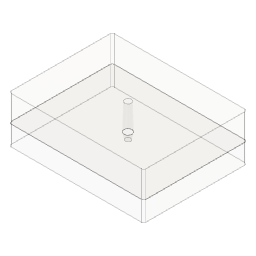
koma (Autodesk Fusion 360 archive; units mm, degrees)
design "MoldSample"
Autodesk Fusion 360 part; units mm, degrees
sketch "スケッチ7" plane through (0, 0, 0) normal (0, 0, 1) x (1, 0, 0)
  line L0 (-40, -25) -> (40, -25)
  line L1 (40, -25) -> (40, 25)
  line L2 (40, 25) -> (-40, 25)
  line L3 (-40, 25) -> (-40, -25)
  line L4 (-40, -25) -> (40, 25) construction
  line L5 (40, -25) -> (-40, 25) construction
  line L6 (-40, 0) -> (40, 0) construction
  line L7 (0, -25) -> (0, 25) construction
  circle A0 centre (-35, 20) radius 2.75
  circle A1 centre (35, 20) radius 2.75
  circle A2 centre (-35, -20) radius 2.75
  circle A3 centre (35, -20) radius 2.75
  line L8 (-29, -23) -> (29, -23)
  line L9 (30, -22) -> (30, 22)
  line L10 (29, 23) -> (-29, 23)
  line L11 (-30, 22) -> (-30, -22)
  line L12 (-30, -23) -> (30, 23) construction
  line L13 (30, -23) -> (-30, 23) construction
  arc A4 (-29, 23) -> (-30, 22) centre (-29, 22) ccw
  arc A5 (30, 22) -> (29, 23) centre (29, 22) ccw
  arc A6 (29, -23) -> (30, -22) centre (29, -22) ccw
  arc A7 (-30, -22) -> (-29, -23) centre (-29, -22) ccw
  circle A8 centre (0, 0) radius 1.5
  arc A9 (-6, 23) -> (6, 23) centre (0, 23) ccw
  arc A10 (-30, -8) -> (-30, 8) centre (-30, 0) ccw
  arc A11 (6, -23) -> (-6, -23) centre (0, -23) ccw
  arc A12 (30, 8) -> (30, -8) centre (30, 0) ccw
  dimension "d41" = 50
  dimension "d42" = 80
  dimension "d43" = 5.5
  dimension "d44" = 5
  dimension "d45" = 5
  dimension "d186" = 46
  dimension "d187" = 10
  dimension "d188" = 1
  dimension "d197" = 3
  dimension "d229" = 8
  dimension "d230" = 6
  constraint horizontal L0
  constraint perpendicular L0 L1
  constraint parallel L0 L2
  constraint parallel L1 L3
  constraint coincident L4 A8.centre
  constraint coincident L5 A8.centre
  constraint coincident A8.centre origin
  constraint midpoint L3 L6.start
  constraint midpoint L1 L6.end
  constraint midpoint L0 L7.start
  constraint midpoint L2 L7.end
  constraint symmetric L7 A0 A1
  constraint symmetric L6 A0 A2
  constraint symmetric L6 A1 A3
  constraint horizontal L8
  constraint perpendicular L8 L9
  constraint parallel L8 L10
  constraint parallel L9 L11
  constraint coincident L12 A8.centre
  constraint coincident L13 A8.centre
  constraint coincident L13.end L11
  constraint coincident L13.end L10
  constraint tangent L11 A4
  constraint tangent L10 A4
  constraint coincident L12.end L10
  constraint coincident L12.end L9
  constraint tangent L10 A5
  constraint tangent L9 A5
  constraint equal A4 A5
  constraint coincident L13.start L9
  constraint coincident L13.start L8
  constraint tangent L9 A6
  constraint tangent L8 A6
  constraint equal A4 A6
  constraint coincident L12.start L8
  constraint coincident L12.start L11
  constraint tangent L8 A7
  constraint tangent L11 A7
  constraint equal A4 A7
  constraint coincident L10 A9.start
  constraint midpoint L10 A9.centre
  constraint coincident L11 A10.start
  constraint midpoint L11 A10.centre
  constraint symmetric L6 A9.start A11.end
  constraint symmetric L6 A9.end A11.start
  constraint symmetric L6 A9 A11
  constraint symmetric L7 A10.start A12.end
  constraint symmetric L7 A10.end A12.start
  constraint symmetric L7 A10 A12
  measures "d41" distance of L0 L2
  measures "d42" distance of L1 L3
  measures "d43" diameter of A0
  measures "d44" distance of L2 A0.centre
  measures "d45" distance of L3 A0.centre
  measures "d186" distance of L8 L10
  measures "d187" distance of L3 L11
  measures "d188" radius of A4
  measures "d197" diameter of A8
  measures "d229" radius of A10
  measures "d230" radius of A9
sketch "Runner" plane through (0, 0, 0) normal (0, 0, 1) x (1, 0, 0)
  line L0 (-14.6, 1.8) -> (-14.6, -1.8)
  arc A0 (-23, -0.6) -> (-21.8, -1.8) centre (-21.8, -0.6) ccw
  line L1 (-17, 1.8) -> (17, 1.8) construction
  line L2 (-14.6, 1.8) -> (-15.4, 3.5)
  line L3 (-17, -3.5) -> (-17, 3.5)
  line L4 (17, 1.8) -> (-17, -1.8) construction
  line L5 (0, 1.8) -> (0, -1.8) construction
  line L6 (-17, 3.5) -> (-15.4, 3.5)
  line L7 (-17, -1.8) -> (-17, 1.8)
  line L8 (-25, -3.5) -> (-9, -3.5) construction
  line L9 (-25.0006, 3.5) -> (-8.9994, 3.5) construction
  arc A1 (21.8, -1.8) -> (23, -0.6) centre (21.8, -0.6) ccw
  line L10 (-17, 1.8) -> (17, -1.8) construction
  line L11 (21.8, -1.8) -> (17, -1.8)
  line L12 (17, 1.8) -> (17, -1.8)
  line L13 (-17, 0) -> (17.3464, 0)
  line L14 (17, 0) -> (23, 0)
  line L15 (-17, 0) -> (-23, 0)
  line L16 (-14.6, -1.8) -> (-15.4, -3.5)
  line L17 (23, 0) -> (23, -0.6)
  line L18 (-17, -3.5) -> (-15.4, -3.5)
  line L19 (-15.4, -3.5) -> (-15.4, 3.5)
  line L20 (17, -1.8) -> (-17, -1.8)
  line L21 (-17, -1.8) -> (-17, 0)
  line L22 (-21.8, -1.8) -> (-17, -1.8)
  line L23 (-23, 0) -> (-23, -0.6)
  circle A2 centre (0, 0) radius 1.8
  circle A3 centre (0, 0) radius 1.5
  dimension "d202" = 1.6
  dimension "d204" = 0.8
  dimension "d210" = 6
  dimension "d211" = 1.2
  dimension "d212" = 3.5
  dimension "d213" = 3.5
  dimension "d214" = 3
  dimension "d215" = 3.6
  dimension "d216" = 17
  constraint horizontal L13
  constraint horizontal L1
  constraint perpendicular L1 L12
  constraint parallel L1 L20
  constraint parallel L7 L12
  constraint coincident A2.centre L10
  constraint coincident A2.centre L4
  constraint midpoint L13.start L7
  constraint vertical L3
  constraint collinear L3 L7
  constraint midpoint L13.start L3
  constraint midpoint L3.end L9
  constraint coincident L2.end L9
  constraint perpendicular L9 L19
  constraint coincident L16.end L8
  constraint coincident L0.end L20
  constraint coincident L16.end L19
  constraint symmetric L0.end L0.start L13
  constraint symmetric L16.end L2.end L13
  constraint horizontal L15
  constraint vertical L23
  constraint horizontal L22
  constraint vertical L21
  constraint collinear L20 L22
  constraint tangent A0 L23
  constraint tangent A0 L22
  constraint midpoint L5.start L1
  constraint midpoint L5.end L20
  constraint symmetric L14.start L13.start L5
  constraint symmetric L15.end L14.end L5
  constraint symmetric L10.end L4.end L5
  constraint symmetric A1.end A0.start L5
  constraint symmetric A1.start A0.end L5
  constraint symmetric A0 L5 A1
  constraint coincident A2.centre A3.centre
  constraint tangent L20 A2
  measures "d202" distance of L3 L19
  measures "d204" distance of L0.end L19
  measures "d210" distance of L3 L23
  measures "d211" radius of A0
  measures "d212" distance of L8 L13
  measures "d213" distance of L9 L13
  measures "d214" diameter of A3
  measures "d215" diameter of A2
  measures "d216" distance of L3 A2.centre
sketch "スケッチ1" plane through (0, 0, 0) normal (0, 0, 1) x (1, 0, 0)
  line L0 (8.5, -3) -> (25.5, -3)
  line L1 (26, -3.5) -> (26, -20.5)
  line L2 (25.5, -21) -> (8.5, -21)
  line L3 (8, -20.5) -> (8, -3.5)
  line L4 (17, -3) -> (17, -21) construction
  line L5 (8, -12) -> (26, -12) construction
  arc A0 (8.5, -3) -> (8, -3.5) centre (8.5, -3.5) ccw
  arc A1 (26, -3.5) -> (25.5, -3) centre (25.5, -3.5) ccw
  arc A2 (25.5, -21) -> (26, -20.5) centre (25.5, -20.5) ccw
  arc A3 (8, -20.5) -> (8.5, -21) centre (8.5, -20.5) ccw
  line L6 (9.7, -4.2) -> (24.3, -4.2)
  line L7 (9.2, -19.3) -> (9.2, -4.7)
  line L8 (24.3, -19.8) -> (9.7, -19.8)
  line L9 (24.8, -4.7) -> (24.8, -19.3)
  arc A4 (9.7, -4.2) -> (9.2, -4.7) centre (9.7, -4.7) ccw
  arc A5 (9.2, -19.3) -> (9.7, -19.8) centre (9.7, -19.3) ccw
  arc A6 (24.3, -19.8) -> (24.8, -19.3) centre (24.3, -19.3) ccw
  arc A7 (24.8, -4.7) -> (24.3, -4.2) centre (24.3, -4.7) ccw
  circle A8 centre (17, -12.03) radius 2.7
  line L10 (14.3525, -11.5) -> (19.6475, -11.5) construction
  line L11 (14.3525, -12.5) -> (19.6475, -12.5) construction
  line L12 (16.5, -9.3767) -> (16.5, -14.6833) construction
  line L13 (17.5, -9.3767) -> (17.5, -14.6833) construction
  line L14 (16.5, -11.5) -> (14.5202, -11.5)
  line L15 (14.5202, -12.5) -> (14.5202, -11.5)
  line L16 (14.5202, -12.5) -> (16.5, -12.5)
  line L17 (15.0202, -11.5) -> (15.0202, -12.5)
  line L18 (16.5, -12.5) -> (16.5, -14.4798)
  line L19 (17.5, -14.4798) -> (17.5, -12.5)
  line L20 (16.5, -13.9798) -> (17.5, -13.9798)
  line L21 (17.5, -14.4798) -> (16.5, -14.4798)
  line L22 (17.5, -12.5) -> (19.4798, -12.5)
  line L23 (19.4798, -11.5) -> (17.5, -11.5)
  line L24 (18.9798, -12.5) -> (18.9798, -11.5)
  line L25 (19.4798, -11.5) -> (19.4798, -12.5)
  line L26 (17.5, -11.5) -> (17.5, -9.5202)
  line L27 (16.5, -9.5202) -> (16.5, -11.5)
  line L28 (17.5, -10.0202) -> (16.5, -10.0202)
  line L29 (16.5, -9.5202) -> (17.5, -9.5202)
  circle A9 centre (13.2, -15.7) radius 1.25
  circle A10 centre (20.8, -15.7) radius 1.25
  point P0 (8, -3)
  point P1 (8, -21)
  point P2 (14.3002, -12)
  point P3 (17, -12)
  dimension "d326" = 18
  dimension "d327" = 18
  dimension "d328" = 8
  dimension "d329" = 3
  dimension "d330" = 0.5
  dimension "d332" = 0.5
  dimension "d333" = 0.03
  dimension "d334" = 5.4
  dimension "d335" = 1.2
  dimension "d336" = 1.2
  dimension "d337" = 1
  dimension "d338" = 1
  dimension "d339" = 0.22
  dimension "d341" = 0.5
  dimension "d343" = 360
  dimension "d366" = 2.5
  dimension "d367" = 12.7
  dimension "d368" = 5.2
  constraint horizontal L0
  constraint vertical L1
  constraint horizontal L2
  constraint vertical L3
  constraint coincident L3 L5.start
  constraint coincident L0 L4.start
  constraint coincident P0 L3
  constraint coincident P0 L0
  constraint tangent L3 A0
  constraint tangent L0 A0
  constraint coincident L1 L5.end
  constraint tangent L0 A1
  constraint tangent L1 A1
  constraint equal A0 A1
  constraint coincident L2 L4.end
  constraint tangent L1 A2
  constraint tangent L2 A2
  constraint equal A0 A2
  constraint coincident P1 L2
  constraint coincident P1 L3
  constraint tangent L2 A3
  constraint tangent L3 A3
  constraint equal A0 A3
  constraint parallel L0 L6
  constraint parallel L3 L7
  constraint parallel L2 L8
  constraint parallel L1 L9
  constraint tangent L6 A4
  constraint tangent L7 A4
  constraint tangent L7 A5
  constraint tangent L8 A5
  constraint equal A4 A5
  constraint tangent L8 A6
  constraint tangent L9 A6
  constraint equal A4 A6
  constraint tangent L9 A7
  constraint tangent L6 A7
  constraint equal A4 A7
  constraint coincident L4 A8.centre
  constraint vertical L4
  constraint horizontal L5
  constraint midpoint L4 L5
  constraint symmetric L5 L6 L8
  constraint symmetric L4 L7 L9
  constraint coincident A8 L10.start
  constraint coincident A8 L10.end
  constraint perpendicular L4 L10
  constraint symmetric L5 L10.start L11.start
  constraint symmetric L5 L10.end L11.end
  constraint coincident A8 L12.start
  constraint coincident A8 L12.end
  constraint vertical L12
  constraint symmetric L4 L12.start L13.start
  constraint symmetric L4 L12.end L13.end
  constraint coincident L10 L14.start
  constraint coincident L12 L14.start
  constraint coincident L10 L14.end
  constraint perpendicular L12 L14
  constraint coincident L11 L15.start
  constraint coincident L12 L16.end
  constraint coincident L11 L16.end
  constraint coincident L5 P2
  constraint coincident A8 P2
  constraint perpendicular L5 L15
  constraint coincident L14 L17.start
  constraint coincident L11 L17.end
  constraint perpendicular L11 L17
  constraint midpoint L4 P3
  constraint symmetric L4 A9 A10
  measures "d326" distance of P0 P1
  measures "d327" distance of L1 L3
  measures "d328" horizontal distance of P0 origin
  measures "d329" vertical distance of P0 origin
  measures "d330" radius of A0
  measures "d332" radius of A4
  measures "d333" distance of L5 A8.centre
  measures "d334" diameter of A8
  measures "d335" distance of L2 L8
  measures "d336" distance of L1 L9
  measures "d337" distance of L10 L11
  measures "d338" distance of L12 L13
  measures "d339" distance of L15 P2
  measures "d341" distance of L15 L17
  measures "d366" diameter of A9
  measures "d367" distance of L0 A9.centre
  measures "d368" distance of L3 A9.centre
ref_plane "作業平面1" through (0, 0, 7.5) normal (0, 0, 1) x (1, 0, 0)
sketch "スケッチ2" plane through (0, 0, 7.5) normal (0, 0, 1) x (1, 0, 0)
  line L0 (8.5, -3) -> (25.5, -3) construction
  line L1 (8, -20.5) -> (8, -3.5) construction
  line L2 (25.5, -21) -> (8.5, -21) construction
  line L3 (26, -3.5) -> (26, -20.5) construction
  arc A0 (26, -3.5) -> (25.5, -3) centre (25.5, -3.5) ccw construction
  arc A1 (8.5, -3) -> (8, -3.5) centre (8.5, -3.5) ccw construction
  arc A2 (8, -20.5) -> (8.5, -21) centre (8.5, -20.5) ccw construction
  arc A3 (25.5, -21) -> (26, -20.5) centre (25.5, -20.5) ccw construction
  line L4 (17, -3) -> (17, -21) construction
  line L5 (8, -12) -> (26, -12) construction
  line L6 (12, -18) -> (22, -18)
  line L7 (23, -17) -> (23, -7)
  line L8 (22, -6) -> (12, -6)
  line L9 (11, -7) -> (11, -17)
  line L10 (11, -18) -> (23, -6) construction
  line L11 (23, -18) -> (11, -6) construction
  arc A4 (12, -6) -> (11, -7) centre (12, -7) ccw
  arc A5 (23, -7) -> (22, -6) centre (22, -7) ccw
  arc A6 (22, -18) -> (23, -17) centre (22, -17) ccw
  arc A7 (11, -17) -> (12, -18) centre (12, -17) ccw
  point P0 (17, -12)
  dimension "d396" = 12
  dimension "d397" = 12
  dimension "d398" = 1
  constraint midpoint L0 L4.start
  constraint midpoint L2 L4.end
  constraint midpoint L1 L5.start
  constraint midpoint L3 L5.end
  constraint horizontal L6
  constraint perpendicular L6 L7
  constraint parallel L6 L8
  constraint parallel L7 L9
  constraint coincident L10 P0
  constraint coincident L11 P0
  constraint midpoint L4 P0
  constraint coincident L11.end L9
  constraint coincident L11.end L8
  constraint tangent L9 A4
  constraint tangent L8 A4
  constraint coincident L10.end L8
  constraint coincident L10.end L7
  constraint tangent L8 A5
  constraint tangent L7 A5
  constraint equal A4 A5
  constraint coincident L11.start L7
  constraint coincident L11.start L6
  constraint tangent L7 A6
  constraint tangent L6 A6
  constraint equal A4 A6
  constraint coincident L10.start L6
  constraint coincident L10.start L9
  constraint tangent L6 A7
  constraint tangent L9 A7
  constraint equal A4 A7
  measures "d396" distance of L7 L9
  measures "d397" distance of L6 L8
  measures "d398" radius of A4
ref_plane "作業平面4" through (0, 0, 6.3) normal (0, 0, 1) x (1, 0, 0)
sketch "スケッチ8" plane through (0, 0, 6.3) normal (0, 0, 1) x (1, 0, 0)
  line L0 (11, -7) -> (11, -17) construction
  line L1 (22, -6) -> (12, -6) construction
  arc A0 (12, -6) -> (11, -7) centre (12, -7) ccw construction
  arc A1 (11, -17) -> (12, -18) centre (12, -17) ccw construction
  line L2 (12, -18) -> (22, -18) construction
  line L3 (23, -17) -> (23, -7) construction
  arc A2 (23, -7) -> (22, -6) centre (22, -7) ccw construction
  arc A3 (22, -18) -> (23, -17) centre (22, -17) ccw construction
  line L4 (21.5, -7) -> (12.5, -7)
  line L5 (12, -7.5) -> (12, -16.5)
  line L6 (12.5, -17) -> (21.5, -17)
  line L7 (22, -16.5) -> (22, -7.5)
  arc A4 (12.5, -7) -> (12, -7.5) centre (12.5, -7.5) ccw
  arc A5 (22, -7.5) -> (21.5, -7) centre (21.5, -7.5) ccw
  arc A6 (21.5, -17) -> (22, -16.5) centre (21.5, -16.5) ccw
  arc A7 (12, -16.5) -> (12.5, -17) centre (12.5, -16.5) ccw
  line L8 (17, -6) -> (17, -18) construction
  line L9 (11, -12) -> (23, -12) construction
  dimension "d400" = 0.5
  dimension "d401" = 1
  dimension "d402" = 1
  constraint parallel L1 L4
  constraint parallel L0 L5
  constraint parallel L2 L6
  constraint parallel L3 L7
  constraint tangent L5 A4
  constraint tangent L4 A4
  constraint tangent L4 A5
  constraint tangent L7 A5
  constraint equal A4 A5
  constraint tangent L7 A6
  constraint tangent L6 A6
  constraint equal A4 A6
  constraint tangent L6 A7
  constraint tangent L5 A7
  constraint equal A4 A7
  constraint midpoint L1 L8.start
  constraint midpoint L2 L8.end
  constraint midpoint L0 L9.start
  constraint midpoint L3 L9.end
  constraint symmetric L5 L7 L8
  constraint symmetric L4 L6 L9
  measures "d400" radius of A4
  measures "d401" distance of L3 L7
  measures "d402" distance of L1 L4
ref_plane "作業平面10" through (0, -12, 0) normal (0, 1, 0) x (0, 0, 1)
sketch "スケッチ28" plane through (0, -12, 0) normal (0, 1, 0) x (1, 0, 0)
  line L0 (17, -7.5) -> (17, 0) construction
  arc A0 (22, -6.3) -> (24.8, 0) centre (7.2558, 4.0252) ccw
  arc A1 (9.2, 0) -> (12, -6.3) centre (26.7442, 4.0252) ccw
  arc A2 (8, 0) -> (11, -7.5) centre (25.7864, 2.7646) ccw
  arc A3 (23, -7.5) -> (26, 0) centre (8.2136, 2.7646) ccw
  point P0 (17, -7.5)
  point P1 (17, 0)
  point P2 (22, -6.3)
  point P3 (12, -6.3)
  point P4 (24.8, 0)
  point P5 (9.2, 0)
  point P6 (11, -7.5)
  point P7 (23, -7.5)
  point P8 (26, 0)
  point P9 (8, 0)
  dimension "d405" = -12
  constraint coincident P0 L0.start
  constraint coincident P1 L0.end
  constraint coincident P4 A0.end
  constraint coincident P2 A0.start
  constraint coincident P5 A1.start
  constraint coincident P3 A1.end
  constraint coincident P9 A2.start
  constraint coincident P6 A2.end
  constraint coincident P8 A3.end
  constraint coincident P7 A3.start
  measures "d411" radius of A1
  measures "d412" radius of A0
  measures "d438" radius of A3
  measures "d439" radius of A2
ref_plane "作業平面11" through (17, -12, 3.75) normal (1, 0, 0) x (0, 0, -1)
ref_plane "作業平面12" through (17, -12, 3.75) normal (0.707107, 0.707107, 0) x (0, 0, -1)
sketch "スケッチ29" plane through (17, -12, 3.6) normal (1, 0, 0) x (0, 1, 0)
  arc A0 (-6, 3.9) -> (-9, -3.6) centre (8.7864, -6.3646) ccw
  line L0 (0, 3.9) -> (-0.03, -3.6)
  arc A1 (9, -3.6) -> (6, 3.9) centre (-8.7864, -6.3646) ccw
  arc A2 (-5, 2.7) -> (-7.8, -3.6) centre (9.7442, -7.6252) ccw
  arc A3 (7.8, -3.6) -> (5, 2.7) centre (-9.7442, -7.6252) ccw
  point P0 (6, 3.9)
  point P1 (-6, 3.9)
  point P2 (-9, -3.6)
  point P3 (0, 3.9)
  point P4 (-0.03, -3.6)
  point P5 (9, -3.6)
  point P6 (-7.8, -3.6)
  point P7 (7.8, -3.6)
  point P8 (-5, 2.7)
  point P9 (5, 2.7)
  dimension "d407" = 18
  dimension "d408" = 18
  dimension "d409" = 18
  dimension "d410" = 18
  constraint coincident P2 A0.end
  constraint coincident P1 A0.start
  constraint coincident P3 L0.start
  constraint coincident P4 L0.end
  constraint coincident P5 A1.start
  constraint coincident P0 A1.end
  constraint coincident P6 A2.end
  constraint coincident P8 A2.start
  constraint coincident P7 A3.start
  constraint coincident P9 A3.end
  measures "d407" radius of A0
  measures "d408" radius of A1
  measures "d409" radius of A2
  measures "d410" radius of A3
sketch "スケッチ27" plane through (0, 0, 0) normal (0, 0, 1) x (1, 0, 0)
  line L0 (8, -20.5) -> (8, -3.5) construction
  line L1 (8.5, -3) -> (25.5, -3) construction
  line L2 (26, -3.5) -> (26, -20.5) construction
  line L3 (25.5, -21) -> (8.5, -21) construction
  arc A0 (8, -20.5) -> (8.5, -21) centre (8.5, -20.5) ccw construction
  arc A1 (8.5, -3) -> (8, -3.5) centre (8.5, -3.5) ccw construction
  arc A2 (25.5, -21) -> (26, -20.5) centre (25.5, -20.5) ccw construction
  arc A3 (26, -3.5) -> (25.5, -3) centre (25.5, -3.5) ccw construction
  line L4 (-29, -23) -> (29, -23) construction
  line L5 (-30, 22) -> (-30, -22) construction
  line L6 (29, 23) -> (-29, 23) construction
  line L7 (30, -22) -> (30, 22) construction
  arc A4 (-29, 23) -> (-30, 22) centre (-29, 22) ccw construction
  arc A5 (-30, -22) -> (-29, -23) centre (-29, -22) ccw construction
  arc A6 (30, 22) -> (29, 23) centre (29, 22) ccw construction
  arc A7 (29, -23) -> (30, -22) centre (29, -22) ccw construction
  line L8 (0, -25) -> (0, 25) construction
  line L9 (-40, 0) -> (40, 0) construction
  line L10 (8, -12) -> (-8, -12) construction
  line L11 (-8, -20.5) -> (-8, -3.5) construction
  line L12 (-8, -16) -> (8, -16) construction
  line L13 (-8, -8) -> (8, -8) construction
  point P0 (8, -12)
  dimension "d387" = 2
  dimension "d388" = 4
  dimension "d389" = 2
  dimension "d390" = 2
  constraint midpoint L0 P0
  constraint perpendicular L0 L10
  constraint symmetric L0.start L8 L11.start
  constraint symmetric L0.end L8 L11.end
  constraint symmetric L8 L10.end P0
  constraint midpoint L10.end L11
  constraint coincident L11 L12.start
  constraint coincident L0 L12.end
  constraint perpendicular L0 L12
  constraint symmetric L10 L12.start L13.start
  constraint symmetric L10 L12.end L13.end
  measures "d388" distance of L10 L12
sketch "スケッチ30" plane through (17, -12, 3.6) normal (0.707107, 0.707107, 0) x (0, 0, -1)
  line L0 (-3.9, -7.7782) -> (-3.9, -8.0711)
  line L1 (-3.9, -0.7071) -> (-3.9, -7.7782)
  line L2 (-3.9, 0.7071) -> (-3.9, -0.7071)
  line L3 (-3.9, 7.7782) -> (-3.9, 0.7071)
  line L4 (-3.9, 8.0711) -> (-3.9, 7.7782)
  line L5 (-2.7, 6.864) -> (-2.7, 6.7175)
  line L6 (-2.7, 6.7175) -> (-2.7, 0.3536)
  line L7 (-2.7, 0.3536) -> (-2.7, -0.3536)
  line L8 (-2.7, -0.3536) -> (-2.7, -6.7175)
  line L9 (-2.7, -6.7175) -> (-2.7, -6.864)
  arc A0 (-3.9, -8.0711) -> (-3.9, 8.0711) centre (-63.3547, 0) ccw
  arc A1 (-2.7, -6.864) -> (-2.7, 6.864) centre (-62.3061, 0) ccw
  line L10 (-3.3547, 0) -> (-3.9, 0)
  line L11 (-2.7, 0) -> (-2.3061, 0)
  dimension "d415" = 60
  dimension "d416" = 60
  constraint coincident L0.end A0.start
  constraint coincident L4.start A0.end
  constraint coincident L9.end A1.start
  constraint coincident L5.start A1.end
  constraint midpoint A0 L10.start
  constraint midpoint L2 L10.end
  constraint midpoint L7 L11.start
  constraint midpoint A1 L11.end
  measures "d415" radius of A1
  measures "d416" radius of A0
extrude "Mold" add sketch "スケッチ7" along normal blind 14 contours L0 L1 L2 L3 | L8 L9 L10 L11 A4 A5 A6 A7 A9 A10 A11 A12 | L8 A11 | L11 A10 | L9 A12 | L10 A9 | A8 makes body 1
extrude "Mold (1)" cut sketch "スケッチ7" along normal blind 12 contours L8 L9 L10 L11 A4 A5 A6 A7 A9 A10 A11 A12 | L8 A11 | L11 A10 | L9 A12 | L10 A9 | A8 bodies 1
extrude "Mold (2)" add sketch "スケッチ7" against normal blind 10.5 separate body contours L0 L1 L2 L3 | L8 L9 L10 L11 A4 A5 A6 A7 A9 A10 A11 A12 | L8 A11 | L11 A10 | L9 A12 | L10 A9 | A8 makes body 2
extrude "押し出し30" cut sketch "スケッチ7" along normal blind 24 contours A8 bodies 1
extrude "Mold (3)" cut sketch "スケッチ7" against normal blind 8.8 contours L8 L9 L10 L11 A4 A5 A6 A7 A9 A10 A11 A12 | L8 A11 | L11 A10 | L9 A12 | L10 A9 | A8 bodies 2
sketch "スケッチ14" plane through (0, 0, 0) normal (0, 1, 0) x (1, 0, 0)
  line L0 (1.2, 3) -> (0, 3)
  line L1 (0, 3) -> (0, 0)
  line L2 (1.5, -14) -> (-1.5, -14)
  line L3 (-1.5, -12) -> (1.5, -12)
  line L4 (0, 0) -> (0, -12)
  line L5 (-1.8, 0) -> (1.8, 0)
  line L6 (1.2, 3) -> (1.8, 0)
  line L7 (1.8, 0) -> (1.5, -12)
  dimension "d218" = 1.2
  dimension "d219" = 3
  constraint coincident L1.end L4.start
  constraint midpoint L3 L4.end
  constraint coincident L5.end L6.end
  constraint coincident L3.end L7.end
  constraint horizontal L0
  constraint vertical L1
  measures "d218" distance of L0.start L1
  measures "d219" distance of L0 L1.end
extrude "押し出し5" add sketch "スケッチ7" against normal blind 8.8 separate body contours L8 L9 L10 L11 A4 A5 A6 A7 A9 A10 A11 A12 | L8 A11 | L11 A10 | L9 A12 | L10 A9 | A8 makes body 3
extrude "押し出し8" add sketch "スケッチ7" along normal blind 11.8 separate body contours L8 L9 L10 L11 A4 A5 A6 A7 A9 A10 A11 A12 | L8 A11 | L11 A10 | L9 A12 | L10 A9 | A8 makes body 4
revolve "回転7" cut sketch "スケッチ14" angle 360 about axis through (0, 0, 1.75) along (0, 0, 1) bodies 3 4
hidden bodies 1 2
equation "d334 = ( 2.7 * 2 ) * 1 mm"
named bodies: "innerMoldBottom", "innerMoldTop", "MoldTop", "MoldBottom", "ejecta_pin_0_017", "ejecta_pin_0_001 (1)", "ejecta_pin_0_020", "ejecta_pin_0_009", "ejecta_pin_0_001", "ejecta_pin_0_018", "ejecta_pin_0_015", "ejecta_pin_0_020 (1)"
